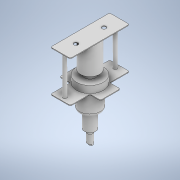
# Autodesk Inventor part: marcadorNUEVO
Saved by Autodesk Inventor 2020 (Build 240168000, 168)
## iProperties
Created: 2022-09-03
Part Number: marcadorNUEVO
Material: Generic
Document SubType Name: Modeling
Designer: robin
Density: 1 g/cm^3
Appearance: Default
Author: robin
Autodesk Inventor part; units mm, degrees
ref_plane "YZ Plane" through (0, 0, 0) normal (1, 0, 0) x (0, 1, 0)
ref_plane "XZ Plane" through (0, 0, 0) normal (0, 1, 0) x (-1, 0, 0)
ref_plane "XY Plane" through (0, 0, 0) normal (0, 0, 1) x (1, 0, 0)
sketch "Sketch1" plane through (0, 0, 0) normal (0, 1, 0) x (-1, 0, 0)
  line L0 (29, 0) -> (29, -12)
  line L1 (27, -14) -> (16, -14)
  line L2 (-16, -14) -> (-27, -14)
  line L3 (-29, -12) -> (-29, 12)
  line L4 (-27, 14) -> (-16, 14)
  line L5 (16, 14) -> (27, 14)
  line L6 (29, 12) -> (29, 0)
  line L7 (14, -16) -> (14, -40)
  line L8 (12, -42) -> (-12, -42)
  line L9 (-14, -40) -> (-14, -16)
  line L10 (-14, 16) -> (-14, 40)
  line L11 (-12, 42) -> (12, 42)
  line L12 (14, 40) -> (14, 16)
  arc A0 (29, 12) -> (27, 14) centre (27, 12) ccw
  arc A1 (27, -14) -> (29, -12) centre (27, -12) ccw
  arc A2 (16, -14) -> (14, -16) centre (16, -16) ccw
  arc A3 (12, -42) -> (14, -40) centre (12, -40) ccw
  arc A4 (-14, -40) -> (-12, -42) centre (-12, -40) ccw
  arc A5 (-14, -16) -> (-16, -14) centre (-16, -16) ccw
  arc A6 (-29, -12) -> (-27, -14) centre (-27, -12) ccw
  arc A7 (-27, 14) -> (-29, 12) centre (-27, 12) ccw
  arc A8 (-16, 14) -> (-14, 16) centre (-16, 16) ccw
  arc A9 (-12, 42) -> (-14, 40) centre (-12, 40) ccw
  arc A10 (14, 40) -> (12, 42) centre (12, 40) ccw
  arc A11 (14, 16) -> (16, 14) centre (16, 16) ccw
  point P0 (0, 0)
  point P1 (29, -14)
  point P2 (14, -14)
  point P3 (-14, -14)
  point P4 (-29, -14)
  point P5 (-29, 14)
  point P6 (-14, 14)
  point P7 (14, -42)
  point P8 (-14, 42)
  point P9 (14, 42)
  dimension "d2" = 14
  dimension "d4" = 15
  dimension "d5" = 28
  dimension "d7" = 28
  dimension "d8" = 28
  dimension "d12" = 2
  constraints: 26 end point, 24 point on circle, 24 tangent, 22 point on line, 12 centre point, 11 equal radius, 7 perpendicular, 1 collinear, 1 vertical
  measures "d2" distance of L0.start point (29, -14)
  measures "d4" distance of point (-14, -14) point (-29, -14)
  measures "d5" distance of point (-29, -14) point (-29, 14)
  measures "d7" distance of point (14, -14) point (14, -42)
  measures "d8" distance of point (-14, 14) point (-14, 42)
  measures "d12" radius of A0
extrude "Extrusion1" add sketch "Sketch1" along normal blind 1
sketch "Sketch2" plane through (0, 1, 0) normal (0, 1, 0) x (1, 0, 0)
  circle A0 centre (0, 0) radius 19
  dimension "d15" = 38
  constraints: 1 centre point, 1 coincident
  measures "d15" diameter of A0
extrude "Extrusion2" add sketch "Sketch2" along normal blind 10
sketch "Sketch3" plane through (0, 11, 0) normal (0, 1, 0) x (1, 0, 0)
  circle A0 centre (0, 0) radius 8
  dimension "d18" = 16
  constraints: 1 centre point, 1 coincident
  measures "d18" diameter of A0
extrude "Extrusion3" add sketch "Sketch3" along normal blind 7
sketch "Sketch4" plane through (0, 18, 0) normal (0, 1, 0) x (1, 0, 0)
  circle A0 centre (0, 0) radius 13.5
  dimension "d21" = 27
  constraints: 1 centre point, 1 coincident
  measures "d21" diameter of A0
extrude "Extrusion4" add sketch "Sketch4" along normal blind 40
sketch "Sketch5" plane through (0, 58, 0) normal (0, 1, 0) x (1, 0, 0)
  line L0 (0, 41.9572) -> (12, 41.9572)
  line L1 (14, 39.9572) -> (14, -40)
  line L2 (12, -42) -> (-12, -42)
  line L3 (-14, -40) -> (-14, 39.9572)
  line L4 (-12, 41.9572) -> (0, 41.9572)
  arc A0 (-12, 41.9572) -> (-14, 39.9572) centre (-12, 39.9572) ccw
  arc A1 (14, 39.9572) -> (12, 41.9572) centre (12, 39.9572) ccw
  arc A2 (12, -42) -> (14, -40) centre (12, -40) ccw
  arc A3 (-14, -40) -> (-12, -42) centre (-12, -40) ccw
  point P0 (0, 0)
  point P1 (-14, 41.9572)
  dimension "d24" = 2
  constraints: 10 end point, 8 point on circle, 8 tangent, 4 centre point, 4 perpendicular, 3 equal radius, 3 point on line, 1 horizontal
  measures "d24" radius of A0
extrude "Extrusion5" add sketch "Sketch5" along normal blind 1
sketch "Sketch6" plane through (0, 1, 0) normal (0, 1, 0) x (1, 0, 0)
  line L0 (0, 0) -> (0, 36)
  line L1 (0, 0) -> (0, -36)
  circle A0 centre (0, 36) radius 2.5
  circle A1 centre (0, -36) radius 2.5
  dimension "d27" = 36
  dimension "d28" = 36
  dimension "d29" = 5
  dimension "d30" = 5
  constraints: 4 end point, 2 centre point, 2 coincident, 2 vertical
  measures "d27" distance of L0.start L0.end
  measures "d28" distance of L0.start L1.end
  measures "d29" diameter of A0
  measures "d30" diameter of A1
extrude "Extrusion6" add sketch "Sketch6" along normal blind 58
sketch "Sketch7" plane through (0, 0, 0) normal (0, -1, 0) x (1, 0, 0)
  circle A0 centre (0, 0) radius 15
  dimension "d33" = 30
  constraints: 1 centre point, 1 coincident
  measures "d33" diameter of A0
extrude "Extrusion7" add sketch "Sketch7" along normal blind 32
sketch "Sketch8" plane through (0, -32, 0) normal (0, -1, 0) x (1, 0, 0)
  circle A0 centre (0, 0) radius 8
  dimension "d36" = 16
  constraints: 1 centre point, 1 coincident
  measures "d36" diameter of A0
extrude "Extrusion8" add sketch "Sketch8" along normal blind 43
fillet "Fillet1" radius 5 1 edges at (-15, -32, 0)
sketch "Sketch9" plane through (0, -75, 0) normal (0, -1, 0) x (1, 0, 0)
  circle A0 centre (0, 0) radius 4
  circle A1 centre (0, 0) radius 12.3979
  dimension "d40" = 8
  constraints: 2 centre point, 2 coincident
  measures "d40" diameter of A0
extrude "Extrusion9" cut sketch "Sketch9" against normal blind 20
fillet "Fillet2" radius 5 1 edges at (-4, -55, 0)
sketch "Sketch10" plane through (14, 0, 40) normal (1, 0, 0) x (0, 0, -1)
  line L0 (36, -75) -> (44, -75) projected
  line L1 (36, -75) -> (38.5, -75)
  line L2 (38.5, -75) -> (38.5, -71.9713)
  line L3 (38.5, -71.9713) -> (36, -71.9713)
  line L4 (36, -71.9713) -> (36, -75)
  line L5 (44, -59.899) -> (44, -75) projected
  line L6 (44, -75) -> (41.5, -75)
  line L7 (41.5, -75) -> (41.5, -71.9713)
  line L8 (41.5, -71.9713) -> (44, -71.9713)
  line L9 (44, -71.9713) -> (44, -75)
  point P0 (40, 0)
  dimension "d44" = 2.5
  dimension "d45" = 2.5
  constraints: 16 end point, 4 parallel, 3 point on line, 2 horizontal, 2 perpendicular
  measures "d44" distance of L3.end L2.end
  measures "d45" distance of L7.end L8.end
extrude "Extrusion10" cut sketch "Sketch10" against normal blind 20
sketch "Sketch11" plane through (-3.7081, -71.9713, 1.5) normal (0, 0, 1) x (1, 0, 0)
  line L0 (7.4162, -3.0287) -> (0, -3.0287) projected
  line L1 (3.7081, -3.0287) -> (8.9248, -1.5011)
  line L2 (8.9248, -1.5011) -> (8.9248, -4.1511)
  line L3 (8.9248, -4.1511) -> (-1.9974, -3.8292)
  line L4 (-1.9974, -3.8292) -> (-1.4278, -1.5011)
  line L5 (-1.4278, -1.5011) -> (3.7081, -3.0287)
  point P0 (3.7081, 71.9713)
  constraints: 10 end point, 1 midpoint, 1 perpendicular
extrude "Extrusion11" cut sketch "Sketch11" against normal blind 20
sketch "Sketch12" plane through (0, 59, 0) normal (0, 1, 0) x (1, 0, 0)
  circle A0 centre (0, 20) radius 3
  circle A1 centre (0, -20) radius 3
  point P0 (0, 0)
  dimension "d51" = 6
  dimension "d52" = 6
  constraints: 2 centre point
  measures "d51" diameter of A0
  measures "d52" diameter of A1
extrude "Extrusion12" cut sketch "Sketch12" against normal blind 20
body "Solid1"
